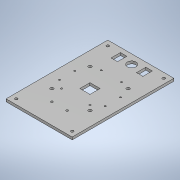
# Autodesk Inventor part: Etage robot réduit
Saved by Autodesk Inventor 2022 (Build 260153000, 153)
## iProperties
Created: 2022-04-26
Part Number: Etage robot réduit
Material: Générique
Document SubType Name: Modeling
Designer: victo
Density: 1 g/cm^3
Appearance: Transparent - Bleu
Author: victo
Autodesk Inventor part; units mm, degrees
ref_plane "YZ Plane" through (0, 0, 0) normal (1, 0, 0) x (0, 1, 0)
ref_plane "XZ Plane" through (0, 0, 0) normal (0, 1, 0) x (-1, 0, 0)
ref_plane "XY Plane" through (0, 0, 0) normal (0, 0, 1) x (1, 0, 0)
sketch "Esquisse1" plane through (0, 0, 0) normal (0, 1, 0) x (-1, 0, 0)
  line L0 (65, -100) -> (-65, -100)
  line L1 (-65, -100) -> (-65, 100)
  line L2 (-65, 100) -> (65, 100)
  line L3 (65, 100) -> (65, -100)
  line L4 (65, -100) -> (-65, 100) construction
  line L5 (-65, -100) -> (65, 100) construction
  circle A0 centre (55, -90) radius 2.6
  line L6 (91, 0) -> (-91, 0) projected
  circle A1 centre (55, 90) radius 2.6
  circle A2 centre (-55, -90) radius 2.6
  circle A3 centre (-55, 90) radius 2.6
  circle A4 centre (0, 0) radius 53.033 construction
  line L7 (-37.5, -37.5) -> (37.5, -37.5) construction
  line L8 (37.5, -37.5) -> (37.5, 37.5) construction
  line L9 (37.5, 37.5) -> (-37.5, 37.5) construction
  line L10 (-37.5, 37.5) -> (-37.5, -37.5) construction
  line L11 (-37.5, -37.5) -> (37.5, 37.5) construction
  line L12 (37.5, -37.5) -> (-37.5, 37.5) construction
  circle A5 centre (37.5, -37.5) radius 3.1
  circle A6 centre (-37.5, -37.5) radius 3.1
  circle A7 centre (-37.5, 37.5) radius 3.1
  circle A8 centre (37.5, 37.5) radius 3.1
  line L13 (-28, -28) -> (28, -28) construction
  line L14 (28, -28) -> (28, 28) construction
  line L15 (28, 28) -> (-28, 28) construction
  line L16 (-28, 28) -> (-28, -28) construction
  line L17 (-28, -28) -> (28, 28) construction
  line L18 (28, -28) -> (-28, 28) construction
  circle A9 centre (28, 28) radius 1.65
  circle A10 centre (-28, 28) radius 1.65
  line L19 (-20, 42) -> (20, 42) construction
  line L20 (20, 42) -> (20, -42) construction
  line L21 (20, -42) -> (-20, -42) construction
  line L22 (-20, -42) -> (-20, 42) construction
  line L23 (-20, 42) -> (20, -42) construction
  line L24 (20, 42) -> (-20, -42) construction
  circle A11 centre (20, -42) radius 1.65
  circle A12 centre (-20, -42) radius 1.65
  circle A13 centre (0, -82) radius 8.5
  line L25 (25, -82) -> (0, -82)
  line L26 (-25, -82) -> (0, -82)
  line L27 (31.35, -91.25) -> (18.65, -91.25)
  line L28 (18.65, -91.25) -> (18.65, -72.75)
  line L29 (18.65, -72.75) -> (31.35, -72.75)
  line L30 (31.35, -72.75) -> (31.35, -91.25)
  line L31 (31.35, -91.25) -> (18.65, -72.75) construction
  line L32 (18.65, -91.25) -> (31.35, -72.75) construction
  line L33 (-31.35, -72.75) -> (-18.65, -72.75)
  line L34 (-18.65, -72.75) -> (-18.65, -91.25)
  line L35 (-18.65, -91.25) -> (-31.35, -91.25)
  line L36 (-31.35, -91.25) -> (-31.35, -72.75)
  line L37 (-31.35, -72.75) -> (-18.65, -91.25) construction
  line L38 (-18.65, -72.75) -> (-31.35, -91.25) construction
  line L39 (0, -140) -> (0, 140) projected
  line L40 (-10, 10) -> (10, 10)
  line L41 (10, 10) -> (10, -10)
  line L42 (10, -10) -> (-10, -10)
  line L43 (-10, -10) -> (-10, 10)
  line L44 (-10, 10) -> (10, -10) construction
  line L45 (10, 10) -> (-10, -10) construction
  line L46 (15, 60) -> (0, 60)
  line L47 (-15, 60) -> (0, 60)
  circle A14 centre (15, 60) radius 2.1
  circle A15 centre (-15, 60) radius 2.1
  line L48 (65, 0) -> (45, 0)
  line L49 (-65, 0) -> (-45, 0)
  line L50 (45, -15) -> (45, 0)
  line L51 (45, 15) -> (45, 0)
  line L52 (-45, -15) -> (-45, 0)
  line L53 (-45, 0) -> (-45, 15)
  circle A16 centre (45, -15) radius 1.65
  circle A17 centre (45, 15) radius 1.65
  circle A18 centre (-45, -15) radius 1.65
  circle A19 centre (-45, 15) radius 1.65
  point P0 (65, -80)
  point P1 (0, 0)
  dimension "d48" = 106.066
  dimension "d1" = 130
  dimension "d2" = 200
  dimension "d8" = 5.2
  dimension "d9" = 10
  dimension "d10" = 10
  dimension "d21" = 10
  dimension "d22" = 10
  dimension "d27" = 10
  dimension "d46" = 6.2
  dimension "d47" = 75
  dimension "d49" = 56
  dimension "d50" = 3.3
  dimension "d51" = 40
  dimension "d52" = 84
  dimension "d53" = 18
  dimension "d54" = 17
  dimension "d55" = 12.7
  dimension "d56" = 18.5
  dimension "d57" = 25
  dimension "d58" = 20
  dimension "d59" = 4.2
  dimension "d60" = 30
  dimension "d61" = 40
  dimension "d62" = 30
  dimension "d63" = 3.3
  dimension "d64" = 20
  constraints: 104 end point, 26 equal length, 19 centre point, 17 midpoint, 15 coincident, 12 point on line, 11 equal radius, 10 perpendicular, 8 horizontal, 2 symmetric about line, 1 vertical, 5 other
  measures "d1" distance of L0.start L0.end
  measures "d2" distance of L0.end L1.end
  measures "d8" diameter of A0
  measures "d9" distance from line of L0 A0.centre
  measures "d10" distance from line of L3 A0.centre
  measures "d21" distance from line of L1 A2.centre
  measures "d22" distance from line of L0 A2.centre
  measures "d27" horizontal distance of point (65, -80) A0.centre
  measures "d46" diameter of A7
  measures "d47" distance of L7.end L8.end
  measures "d49" distance of L14.end L15.end
  measures "d50" diameter of A9
  measures "d51" distance of L20.end L21.end
  measures "d52" distance of L19.end L20.end
  measures "d53" distance between parallel lines of L26 L0
  measures "d54" diameter of A13
  measures "d55" distance of L27.start L27.end
  measures "d56" distance of L29.end L27.start
  measures "d57" distance of L26.start L25.end
  measures "d58" distance of L41.end L42.end
  measures "d59" diameter of A14
  measures "d60" distance of L47.start L46.start
  measures "d61" distance between parallel lines of L2 L46
  measures "d62" distance of L51.start L50.start
  measures "d63" diameter of A16
  measures "d64" distance of L49.start L49.end
extrude "Extrusion1" add sketch "Esquisse1" against normal blind 5 contours L0 L39 A13 L42 L41 L6 L3 | L0 L1 L6 L43 L42 L39 A13 | L6 L41 L40 L39 L2 L3 | L1 L2 L39 L40 L43 L6
